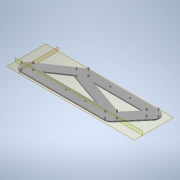
# Autodesk Inventor part: Kogel houders
Saved by Autodesk Inventor 2021 (Build 250183000, 183)
## iProperties
Manager: PJ / DCS
Company: Emmaüs Bovenbouw Aalter
Created: 2021-03-07
Part Number: Kogel houders
Material: S235
Catalog Web Link: http://emmausbovenbouw.op-weg.be/
Vendor: Emmaüsinstituut Bovenbouw Aalter
Document SubType Name: Modeling
Designer: Antho
Engineer: Declercq St.
Manufacturer: Standard
Standards Organization: Custom
Density: 7.86 g/cm^3
Appearance: Steel
Title: Algemene titel
Subject: Specifieke titel
Author: Antho
Keywords: Ruwe Ø xxxxx
Comments: Opmerking
Autodesk Inventor part; units mm, degrees
sketch "Sketch1" plane through (0, 0, 0) normal (0, 0, 1) x (1, 0, 0)
  line L0 (0, 19.7393) -> (0, -19.7393) construction
  line L1 (-39.8995, 0) -> (39.8995, 0) construction
  line L2 (0, 0) -> (191.205, 0)
  line L3 (191.205, 0) -> (235.078, 0)
  line L4 (235.078, 0) -> (235.078, 51)
  line L5 (235.078, 51) -> (191.205, 0)
  line L6 (235.078, 51) -> (74.794, 51)
  line L7 (74.794, 51) -> (0, 0)
  circle A0 centre (0, 0) radius 15
  circle A1 centre (74.794, 51) radius 15
  circle A2 centre (235.078, 51) radius 15
  circle A3 centre (191.205, 0) radius 15
  line L8 (0, -15) -> (191.205, -15)
  line L9 (66.3435, 63.3931) -> (-8.4505, 12.3931)
  line L10 (235.078, 66) -> (74.794, 66)
  line L11 (246.4493, 41.2177) -> (202.5763, -9.7823)
  line L12 (89.794, 51) -> (196.1144, 14.1738)
  line L13 (67.4995, 37.8931) -> (176.2071, 0.2497)
  line L14 (67.4995, 37.8931) -> (182.5402, 37.8931) construction
  line L15 (12.3931, 8.4505) -> (152.5246, 8.4505)
  line L16 (191.205, 15.8743) -> (240.505, 15.8743) construction
  line L17 (191.205, 15.8743) -> (220.1505, 49.5266)
  line L18 (191.205, 15.8743) -> (235.5933, 15.8743) construction
  line L19 (67.4995, 37.8931) -> (24.3222, 8.4505)
  line L20 (67.4995, 37.8931) -> (119.76, 37.8931) construction
  line L21 (217.3382, 46.2569) -> (89.0244, 46.2569)
  line L22 (217.3382, 46.2569) -> (345.652, 46.2569) construction
  point P0 (220.078, 51)
  point P1 (225.2957, 39.6287)
  point P2 (200.9873, 11.3713)
  point P3 (176.205, 0)
  point P4 (15, 0)
  point P5 (12.3931, 8.4505)
  point P6 (62.4009, 42.5495)
  point P7 (103.4876, 46.2569)
  dimension "d0" = 191.205
  dimension "d1" = 43.873
  dimension "d2" = 51
  dimension "d3" = 160.284
  dimension "d4" = 30
  dimension "d5" = 30
  dimension "d6" = 30
  dimension "d7" = 30
  dimension "d8" = 19.1
  dimension "d44" = 49.3
  dimension "d45" = 145.71
  dimension "d46" = 180
  constraints: 46 end point, 15 point on circle, 9 horizontal, 7 point on line, 6 tangent, 5 coincident, 4 centre point, 4 equal length, 2 midpoint, 2 vertical, 1 parallel
  measures "d0" distance of L2.start L2.end
  measures "d1" distance of L2.end L3.end
  measures "d2" distance of L3.end L4.end
  measures "d3" distance of L4.end L6.end
  measures "d4" diameter of A0
  measures "d5" diameter of A1
  measures "d6" diameter of A2
  measures "d7" diameter of A3
  measures "d8" angle of L13 L14
  measures "d44" angle of L18 L17
  measures "d45" angle of L19 L20
  measures "d46" angle of L21 L22
extrude "Extrusion1" add sketch "Sketch1" along normal blind 3 contours L7 A0 L2 | L2 A0 L7 | A0 L15 L13 A3 L2 | L2 A3 L8 A0 | A0 L9 A1 L7 | L7 A1 L19 L15 | A3 L5 L2 | L2 L3 A3 | A1 L6 L7 | L7 L6 A1 L13 | L5 A3 L3 | L13 A1 L21 L12 A3 | A3 L5 A2 L4 L11 L3 | L3 L11 A3 | A3 L12 L17 A2 L5 | A1 L10 A2 L6 | L12 L21 A1 | L6 A2 L17 L21 L12 | A2 L6 L5 | L5 L4 A2 | A2 L4 L6 | L4 A2 L11
sketch "Sketch2" plane through (0, 0, 3) normal (0, 0, 1) x (1, 0, 0)
  arc A0 (-8.4505, 12.3931) -> (0, -15) centre (0, 0) ccw projected
  circle A1 centre (0, 0) radius 15
  line L0 (0, 15) -> (0, 13.5)
  circle A2 centre (0, 0) radius 13.5
  circle A3 centre (0, 13.5) radius 1.5
  circle A4 centre (13.5, 0) radius 1.5
  circle A5 centre (0, -13.5) radius 1.5
  circle A6 centre (-13.5, 0) radius 1.5
  arc A7 (246.4493, 41.2177) -> (235.078, 66) centre (235.078, 51) ccw projected
  circle A8 centre (235.078, 51) radius 13.5
  circle A9 centre (235.078, 64.5) radius 1.5
  circle A10 centre (248.578, 51) radius 1.5
  circle A11 centre (235.078, 37.5) radius 1.5
  circle A12 centre (221.578, 51) radius 1.5
  arc A13 (191.205, -15) -> (202.5763, -9.7823) centre (191.205, 0) ccw projected
  circle A14 centre (191.205, 0) radius 13.5
  circle A15 centre (191.205, 13.5) radius 1.5
  circle A16 centre (204.705, 0) radius 1.5
  circle A17 centre (191.205, -13.5) radius 1.5
  circle A18 centre (177.705, 0) radius 1.5
  arc A19 (74.794, 66) -> (66.3435, 63.3931) centre (74.794, 51) ccw projected
  circle A20 centre (74.794, 51) radius 13.5
  circle A21 centre (74.794, 64.5) radius 1.5
  circle A22 centre (88.294, 51) radius 1.5
  circle A23 centre (74.794, 37.5) radius 1.5
  circle A24 centre (61.294, 51) radius 1.5
  dimension "d11" = 1.5
  dimension "d12" = 3
  dimension "d13" = 3
  dimension "d14" = 27
  dimension "d15" = 3
  dimension "d16" = 3
  dimension "d17" = 3
  dimension "d18" = 3
  dimension "d19" = 27
  dimension "d20" = 3
  dimension "d21" = 3
  dimension "d22" = 3
  dimension "d23" = 3
  dimension "d24" = 27
  dimension "d25" = 3
  dimension "d26" = 3
  dimension "d27" = 3
  dimension "d28" = 3
  constraints: 21 centre point, 18 point on circle, 6 coincident, 2 end point, 1 vertical
  measures "d11" distance of L0.start L0.end
  measures "d12" diameter of A3
  measures "d13" diameter of A5
  measures "d14" diameter of A8
  measures "d15" diameter of A9
  measures "d16" diameter of A10
  measures "d17" diameter of A11
  measures "d18" diameter of A12
  measures "d19" diameter of A14
  measures "d20" diameter of A15
  measures "d21" diameter of A16
  measures "d22" diameter of A17
  measures "d23" diameter of A18
  measures "d24" diameter of A20
  measures "d25" diameter of A21
  measures "d26" diameter of A22
  measures "d27" diameter of A23
  measures "d28" diameter of A24
extrude "Extrusion2" add sketch "Sketch2" along normal blind 5 contours A6 A2 | A3 A2 L0 | L0 A2 A3 | A5 A2 | A6 A2 | A4 A2 | A2 A3 | A5 A2 | A2 A4 | A10 A8 | A9 A8 | A8 A10 | A8 A9 | A11 A8 | A8 A11 | A12 A8 | A8 A12 | A14 A16 | A14 A16 | A15 A14 | A14 A15 | A17 A14 | A14 A17 | A18 A14 | A14 A18 | A20 A22 | A20 A22 | A21 A20 | A20 A21 | A23 A20 | A20 A23 | A24 A20 | A20 A24
sketch "Sketch3" plane through (0, 0, 3) normal (0, 0, 1) x (1, 0, 0)
  line L0 (0, 0) -> (88.434, 0)
  line L1 (176.205, 0) -> (15, 0) projected
  line L2 (88.434, 0) -> (137.2649, 0)
  line L3 (88.434, 0) -> (133.205, 0)
  line L4 (133.205, 0) -> (133.205, 56.318)
  line L5 (133.205, 56.318) -> (177.976, 56.318)
  dimension "d31" = 88.434
  dimension "d32" = 44.771
  dimension "d33" = 56.318
  dimension "d34" = 44.771
  constraints: 10 end point, 4 coincident, 3 point on line, 1 horizontal, 1 vertical
  measures "d31" distance of L0.start L0.end
  measures "d32" distance of L0.end L3.end
  measures "d33" distance of L3.end L4.end
  measures "d34" distance of L4.end L5.end
hole "Hole1" at (88.434, 0, 3) at (133.205, 0, 3) at (133.205, 56.318, 3) at (177.976, 56.318, 3) direction (0, 0, -1) diameter 4.2 depth 5
body "Solid1"
